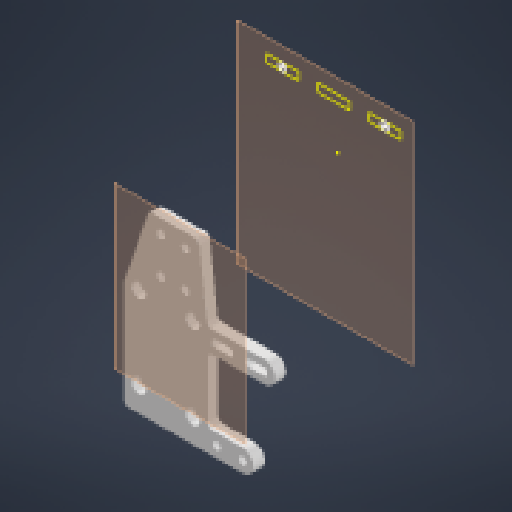
# Autodesk Inventor part: rails-bolts
Saved by Autodesk Inventor 2025 (Build 290162000, 162)
## iProperties
Created: 2024-07-18
Part Number: rails-bolts
Material: Generic
Document SubType Name: Modeling
Designer: Windows 7 was better
Density: 1 g/cm^3
Appearance: Default
Author: Windows 7 was better
Autodesk Inventor part; units mm, degrees
ref_plane "YZ Plane" through (0, 0, 0) normal (1, 0, 0) x (0, 1, 0)
ref_plane "XZ Plane" through (0, 0, 0) normal (0, 1, 0) x (-1, 0, 0)
ref_plane "XY Plane" through (0, 0, 0) normal (0, 0, 1) x (1, 0, 0)
ref_plane "Work Plane1" through (-1.6596, -28.9901, 28.1919) normal (0, 0, 1) x (1, 0, 0)
sketch "Sketch1" plane through (-1.6596, -28.9901, 28.1919) normal (0, 0, 1) x (1, 0, 0)
  spline S0 degree 3 poles (-18.1261, -96.0287) (-18.1261, -96.0287) (-18.0932, -96.0287) (-18.0298, -96.0287) (-17.8251, -96.0287) (-17.2794, -96.0287) (-16.7467, -96.0287) (-16.213, -96.0287) (-15.7353, -96.0287) (-15.6244, -96.0287) (-15.6063, -96.0287) (-15.5971, -96.0287) (-15.5971, -96.0287) knots 0.499993 0.499993 0.499993 0.499993 0.562494 0.562494 0.562494 0.764477 0.764477 0.764477 0.966846 0.966846 0.966846 1 1 1 1 construction
  line L0 (-18.3185, -96.0287) -> (-15.9665, -96.0287) construction
  arc A0 (-13.8616, 2.5089) -> (-19.8616, 2.5089) centre (-16.8616, 2.5089) ccw construction
  arc A1 (-13.9993, -31.5037) -> (-19.9993, -31.5037) centre (-16.9993, -31.5037) ccw construction
  arc A2 (3.0015, -1.5044) -> (9.0015, -1.5044) centre (6.0015, -1.5044) ccw
  circle A3 centre (-16.8616, -31.5037) radius 1.6
  circle A4 centre (5.3371, -31.5037) radius 1.6
  circle A5 centre (-16.8616, 2.5089) radius 1.6
  circle A6 centre (5.3371, 2.5089) radius 1.6
  line L1 (-19.8616, 2.5089) -> (-22.8616, 2.5089) construction
  line L2 (6.9371, 2.5089) -> (11.3371, 2.5089) construction
  line L3 (-16.8616, -33.1037) -> (-16.8616, -36.2364) construction
  line L4 (-12.7018, 32.5036) -> (-22.8616, 2.5089)
  line L5 (-22.8616, 2.5089) -> (-22.8616, -36.2364)
  line L6 (7.9619, 32.5036) -> (11.3371, 2.5089)
  line L7 (11.3371, 2.5089) -> (11.3371, -36.2364)
  line L8 (11.3371, -36.2364) -> (-22.8616, -36.2364)
  line L9 (2.3051, 26.8467) -> (7.9619, 32.5036) construction
  line L10 (-12.7018, 32.5036) -> (7.9619, 32.5036)
  line L11 (2.3051, 26.8467) -> (-7.6949, 26.8467) construction
  line L12 (-19.8616, 78.2844) -> (-2.5116, 78.2844) construction
  line L13 (-11.1866, 78.2844) -> (-4.9166, 78.2844) construction
  line L14 (-11.1866, 78.2844) -> (-17.4566, 78.2844) construction
  line L15 (-19.8616, 78.2844) -> (-17.4566, 78.2844) construction
  line L16 (-4.9166, 78.2844) -> (-2.5116, 78.2844) construction
  line L17 (-7.6949, 26.8467) -> (-7.6949, 11.8467) construction
  circle A7 centre (-7.6949, 26.8467) radius 1.6
  circle A8 centre (-7.6949, 11.8467) radius 1.6
  line L18 (-7.6949, 11.8467) -> (2.3051, 11.8467) construction
  circle A9 centre (2.3051, 11.8467) radius 1.6
  circle A10 centre (2.3051, 26.8467) radius 1.6
  point P0 (1.6596, 28.9901)
  point P1 (-18.3185, 3.0171)
  point P2 (-15.9662, 3.4042)
  dimension "d5" = 3.2
  dimension "d8" = 3.2
  dimension "d6" = 3.2
  dimension "d7" = 3.2
  dimension "d51" = 3
  dimension "d52" = 4.4
  dimension "d56" = 8
  dimension "d58" = 10
  dimension "d59" = 17.35
  dimension "d60" = 6.27
  dimension "d61" = 6.27
  dimension "d62" = 15
  dimension "d63" = 3.2
  dimension "d64" = 3.2
  dimension "d65" = 3.2
  dimension "d66" = 3.2
  constraints: 38 end point, 9 centre point, 6 point on circle, 5 coincident, 5 horizontal, 4 vertical, 2 collinear, 2 point on line, 1 horizontal alignment, 1 midpoint, 1 perpendicular, 1 vertical alignment, 24 other
  measures "d6" diameter of A4
  measures "d7" diameter of A5
  measures "d51" distance of L1.start L1.end
  measures "d52" distance of L2.start L2.end
  measures "d56" distance of L9.start L6.start
  measures "d58" distance of L9.start L11.end
  measures "d59" distance of L12.start L12.end
  measures "d60" distance of L13.start L13.end
  measures "d61" distance of L13.start L14.end
  measures "d62" distance of L11.end L17.end
  measures "d63" diameter of A7
  measures "d64" diameter of A8
  measures "d65" diameter of A9
  measures "d66" diameter of A10
ref_plane "Work Plane2" through (-8.6352, -23.8919, -35.0523) normal (0, 0, 1) x (1, 0, 0)
sketch "Sketch2" plane through (-8.6352, -23.8919, -35.0523) normal (0, 0, 1) x (1, 0, 0)
  line L0 (-7.5414, 41.3535) -> (-20.5414, 41.3535) projected
  line L1 (-20.5414, 44.5535) -> (-7.5414, 44.5535) projected
  line L2 (-7.5414, 44.5535) -> (-7.5414, 41.3535) projected
  line L3 (-20.5414, 41.3535) -> (-20.5414, 44.5535) projected
  line L4 (13.5, 41.3535) -> (0.5, 41.3535) projected
  line L5 (0.5, 44.5535) -> (13.5, 44.5535) projected
  line L6 (13.5, 44.5535) -> (13.5, 41.3535) projected
  line L7 (0.5, 41.3535) -> (0.5, 44.5535) projected
  line L8 (34.55, 41.3535) -> (21.55, 41.3535) projected
  line L9 (21.55, 44.5535) -> (34.55, 44.5535) projected
  line L10 (21.55, 41.3535) -> (21.55, 44.5535) projected
  line L11 (34.55, 44.5535) -> (34.55, 41.3535) projected
  line L12 (-14.0414, 44.5535) -> (-14.0414, 41.3535) construction
  line L13 (28.05, 44.5535) -> (28.05, 41.3535) construction
  circle A0 centre (-14.0414, 42.9535) radius 1.6
  circle A1 centre (28.05, 42.9535) radius 1.6
  point P0 (8.6352, 23.8919)
  constraints: 6 midpoint, 4 end point, 2 vertical alignment, 4 other
extrude "Extrusion1" add sketch "Sketch1" against normal blind 4.5
sketch "Sketch3" plane through (-1.6596, -28.9901, 28.1919) normal (0, 0, 1) x (1, 0, 0)
  line L0 (19.4071, -58.7998) -> (21.4071, -58.7998) construction
  line L1 (20.4071, -58.7998) -> (20.4979, -36.9098) construction
  line L2 (20.4979, -36.9098) -> (25.7879, -36.9098) construction
  line L3 (25.7879, -36.9098) -> (15.2079, -36.9098) construction
  circle A0 centre (15.2079, -36.9098) radius 1.6
  circle A1 centre (25.7879, -36.9098) radius 1.6
  circle A2 centre (15.2079, -36.9098) radius 4.6
  circle A3 centre (25.7879, -36.9098) radius 4.6
  line L4 (25.7879, -32.3098) -> (9.0007, -32.3098)
  line L5 (9.0007, -34.5533) -> (9.0007, 32.4467) projected
  line L6 (25.7879, -41.5098) -> (15.2079, -41.5098)
  line L7 (15.2079, -41.5098) -> (-19.9993, -41.5098)
  line L8 (-19.9993, -34.5533) -> (-19.9993, 32.4467) projected
  line L9 (-19.9993, -41.5098) -> (-19.9993, -34.5533)
  line L10 (-19.9993, -34.5533) -> (9.0007, -34.5533)
  line L11 (9.0007, -34.5533) -> (9.0007, -32.3098)
  line L12 (25.7879, -36.9098) -> (30.1497, -38.3706)
  line L13 (45.9071, 7.0963) -> (8.7371, 7.0963) construction
  line L14 (8.7371, 7.0963) -> (14.7371, 7.0963) construction
  line L15 (14.7371, 7.0963) -> (14.7371, -0.9037) construction
  line L16 (14.7371, -0.9037) -> (34.7371, -0.9037) construction
  line L17 (14.7371, -0.9037) -> (20.7371, -0.9037) construction
  line L18 (14.7371, -2.4037) -> (20.7371, -2.4037)
  line L19 (20.7371, 0.5963) -> (14.7371, 0.5963)
  arc A4 (14.7371, 0.5963) -> (14.7371, -2.4037) centre (14.7371, -0.9037) ccw
  arc A5 (20.7371, -2.4037) -> (20.7371, 0.5963) centre (20.7371, -0.9037) ccw
  line L20 (34.7371, -0.9037) -> (28.7371, -0.9037) construction
  line L21 (34.7371, 0.5963) -> (28.7371, 0.5963)
  line L22 (28.7371, -2.4037) -> (34.7371, -2.4037)
  arc A6 (34.7371, -2.4037) -> (34.7371, 0.5963) centre (34.7371, -0.9037) ccw
  arc A7 (28.7371, 0.5963) -> (28.7371, -2.4037) centre (28.7371, -0.9037) ccw
  line L23 (34.7371, 3.5963) -> (28.7371, 3.5963)
  arc A8 (28.7371, 3.5963) -> (28.7371, -5.4037) centre (28.7371, -0.9037) ccw
  line L24 (28.7371, -5.4037) -> (34.7371, -5.4037)
  arc A9 (34.7371, -5.4037) -> (34.7371, 3.5963) centre (34.7371, -0.9037) ccw
  line L25 (28.7371, 3.5963) -> (9.0007, 3.5963)
  line L26 (28.7371, -5.4037) -> (9.0007, -5.4037)
  line L27 (11.3371, -36.2364) -> (-22.8616, -36.2364) projected
  line L28 (-22.8616, -36.2364) -> (-22.8616, -41.5098)
  line L29 (-22.8616, -41.5098) -> (-19.9993, -41.5098)
  point P0 (1.6596, 28.9901)
  point P1 (11.4479, -23.0098)
  point P2 (9.0007, -15.5098)
  point P3 (17.7371, -0.9037)
  point P4 (31.7371, -0.9037)
  point P5 (-19.9993, -36.2364)
  dimension "d9" = 10.58
  dimension "d10" = 5.29
  dimension "d11" = 10.58
  dimension "d12" = 3.2
  dimension "d13" = 3.2
  dimension "d14" = 3
  dimension "d15" = 3
  dimension "d43" = 6
  dimension "d44" = 8
  dimension "d45" = 20
  dimension "d46" = 6
  dimension "d47" = 3
  dimension "d48" = 6
  dimension "d49" = 3
  dimension "d50" = 3
  constraints: 58 end point, 15 point on circle, 9 centre point, 9 tangent, 8 point on line, 7 perpendicular, 5 horizontal, 4 parallel, 3 midpoint, 2 coincident, 2 collinear, 1 vertical, 1 vertical alignment, 12 other
  measures "d9" distance of L3.end L2.end
  measures "d10" distance of L1.end L2.end
  measures "d11" distance of L2.end L3.end
  measures "d12" diameter of A0
  measures "d13" diameter of A1
  measures "d15" radial gap between concentric circles of A1 A3
  measures "d43" distance of L13.end L14.end
  measures "d44" distance of L14.end L15.end
  measures "d45" distance of L15.end L16.end
  measures "d46" distance of L15.end L17.end
  measures "d47" diameter of A5
  measures "d48" distance of L16.end L20.end
  measures "d49" diameter of A7
  measures "d50" radial gap between concentric circles of A6 A9
extrude "Extrusion2" add sketch "Sketch3" against normal blind 4.5
sketch "Sketch4" plane through (-1.6596, -28.9901, 23.6919) normal (0, 0, -1) x (-1, 0, 0)
  circle A0 centre (-2.3051, 26.8467) radius 1.6 projected
  circle A1 centre (-2.3051, 26.8467) radius 3
  circle A2 centre (7.6949, 26.8467) radius 1.6 projected
  circle A3 centre (7.6949, 26.8467) radius 3
  circle A4 centre (7.6949, 11.8467) radius 1.6 projected
  circle A5 centre (7.6949, 11.8467) radius 3
  circle A6 centre (-2.3051, 11.8467) radius 1.6 projected
  circle A7 centre (-2.3051, 11.8467) radius 3
  dimension "d67" = 6
  dimension "d68" = 6
  dimension "d69" = 6
  dimension "d70" = 6
  constraints: 4 centre point, 4 coincident
  measures "d67" diameter of A1
  measures "d68" diameter of A3
  measures "d69" diameter of A5
  measures "d70" diameter of A7
extrude "Extrusion3" cut sketch "Sketch4" against normal blind 3.5
fillet "Fillet1" radius 2 7 edges at (-24.5212, -70.4999, 25.9419) (9.6775, -34.3938, 25.9419) (9.6775, -61.2999, 25.9419) (9.5552, -25.3938, 25.9419) (-14.3614, 3.5135, 25.9419) (6.3023, 3.5135, 25.9419) (-24.5212, -26.4812, 25.9419)
sketch "Sketch5" plane through (-1.6596, -28.9901, 28.1919) normal (0, 0, 1) x (1, 0, 0)
  circle A0 centre (-16.8616, 2.5089) radius 1.6 projected
  circle A1 centre (-16.8616, 2.5089) radius 3
  circle A2 centre (5.3371, 2.5089) radius 1.6 projected
  circle A3 centre (5.3371, 2.5089) radius 3
  circle A4 centre (-16.8616, -31.5037) radius 1.6 projected
  circle A5 centre (-16.8616, -31.5037) radius 3
  circle A6 centre (5.3371, -31.5037) radius 1.6 projected
  circle A7 centre (5.3371, -31.5037) radius 3
  point P0 (1.6596, 28.9901)
  dimension "d25" = 6
  dimension "d26" = 6
  dimension "d27" = 6
  dimension "d28" = 6
  constraints: 4 centre point, 4 coincident
  measures "d25" diameter of A1
  measures "d26" diameter of A3
  measures "d27" diameter of A5
  measures "d28" diameter of A7
extrude "Extrusion4" cut sketch "Sketch5" against normal blind 3.5 contours A1 | A2 | A3 | A5 | A7
body "Solid1"
